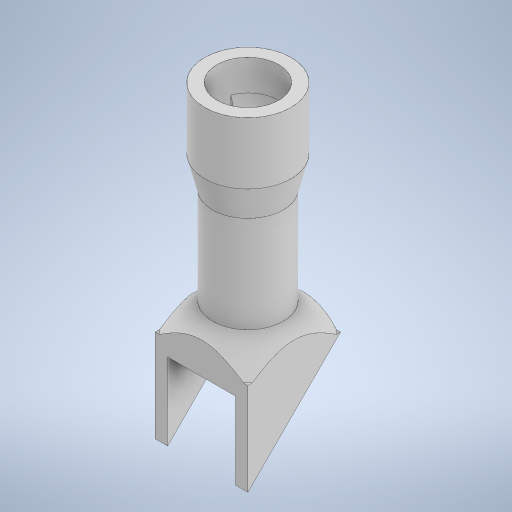
# Autodesk Inventor part: LD to Mirror path
Saved by Autodesk Inventor 2024 (Build 280153000, 153)
## iProperties
Created: 2024-10-15
Part Number: LD to Mirror path
Material: Generic
Document SubType Name: Modeling
Designer: Williamow
Density: 1 g/cm^3
Appearance: Default
Author: Williamow
Autodesk Inventor part; units mm, degrees
ref_plane "YZ Plane" through (0, 0, 0) normal (1, 0, 0) x (0, 1, 0)
ref_plane "XZ Plane" through (0, 0, 0) normal (0, 1, 0) x (-1, 0, 0)
ref_plane "XY Plane" through (0, 0, 0) normal (0, 0, 1) x (1, 0, 0)
sketch "Sketch1" plane through (0, 0, 0) normal (0, 1, 0) x (-1, 0, 0)
  line L0 (3, 3) -> (-3, 3)
  line L1 (-3, 3) -> (-3, -3)
  line L2 (-3, -3) -> (3, -3)
  line L3 (3, -3) -> (3, 3)
  arc A0 (1.299, 0.75) -> (1.299, -0.75) centre (0, 0) ccw
  arc A1 (2.1743, 0.75) -> (2.1743, -0.75) centre (0, 0) ccw
  line L4 (1.299, 0.75) -> (2.1743, 0.75)
  line L5 (1.299, -0.75) -> (2.1743, -0.75)
  circle A2 centre (0, 0) radius 0.2
  line L6 (2.2, 3) -> (2.2, -3)
  line L7 (-2.2, 3) -> (-2.2, -3)
  point P0 (0, -3)
  point P1 (3, 0)
  dimension "d0" = 6
  dimension "d1" = 1.5
  dimension "d2" = 0.8
  dimension "d3" = 1.5
  dimension "d4" = 0.4
  dimension "d5" = 0.8
  dimension "d6" = 0.8
  constraints: 16 end point, 4 point on circle, 4 point on line, 3 centre point, 3 coincident, 3 parallel, 3 perpendicular, 2 equal length, 2 horizontal, 2 midpoint, 1 horizontal alignment, 1 vertical alignment
  measures "d0" distance of L0.start L0.end
  measures "d1" radius of A0
  measures "d2" radial gap between concentric circles of A1 A0
  measures "d3" distance between parallel lines of L5 L4
  measures "d4" diameter of A2
  measures "d5" distance between parallel lines of L1 L7
  measures "d6" distance between parallel lines of L3 L6
extrude "Extrusion1" add sketch "Sketch1" against normal blind 1
extrude "Extrusion2" add sketch "Sketch1" along normal blind 10 contours L7 A1 | A1 L4 A0 L5 L7
extrude "Extrusion3" add sketch "Sketch1" against normal blind 6 contours L3 L2 L6 L0 | L7 A1 L2 L1 L0 | L7 A1
chamfer "Chamfer1" distance 6 angle 45 2 edges at (2.6, -6, -3) (-2.6, -6, -3)
chamfer "Chamfer2" distance 1.75 angle 45 1 edges at (2.3, 0, 0)
sketch "Sketch2" plane through (0, 10, 0) normal (0, 1, 0) x (1, 0, 0)
  circle A0 centre (0, 0) radius 0.2 projected
  circle A1 centre (0, 0) radius 2
  circle A2 centre (0, 0) radius 2.8
  dimension "d19" = 4
  dimension "d20" = 0.8
  constraints: 2 centre point, 2 coincident
  measures "d19" diameter of A1
  measures "d20" radial gap between concentric circles of A1 A2
extrude "Extrusion4" add sketch "Sketch2" along normal blind 4 contours A2
chamfer "Chamfer3" distance 0.5 distance2 2 2 edges at (0.382, 10, -1.9632) (0.382, 10, 1.9632) measured on face at (0.3629, 10, -1.865) measured on face at (0.3629, 10, 1.865)
chamfer "Chamfer4" distance 0.5 distance2 2 1 edges at (2.3, 10, 0) measured on face at (2.4, 10, 0)
body "Solid1"
